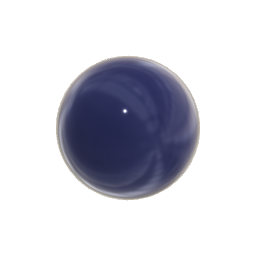
lab0_design v1 (Autodesk Fusion 360 design; units mm, degrees)
Autodesk Fusion 360 part; units mm, degrees
sketch "Sketch1" plane through (0, 0, 0) normal (0, 0, 1) x (1, 0, 0)
  line L0 (0, 10) -> (0, 8)
  line L1 (0, -8) -> (0, -10)
  arc A0 (0, -10) -> (0, 10) centre (0, 0) ccw
  arc A1 (0, -8) -> (0, 8) centre (0, 0) ccw
  dimension "d2" = 10
  constraint coincident A0.centre A1.centre
  constraint vertical L0
  constraint collinear L0 L1
  measures "d2" radius of A0
revolve "Revolve1" add sketch "Sketch1" angle 360 about axis through (0, 1.75, 0) along (0, 1, 0)
